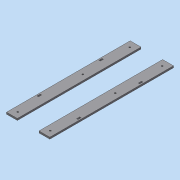
# Autodesk Inventor part: axis-holder_front-front
Saved by Autodesk Inventor 2016 SP1 (Build 200210100, 210)
## iProperties
Created: 2016-03-25
Part Number: axis-holder_front-front
Material: Generic
Document SubType Name: Modeling
Designer: Mohamed A.
Density: 1 g/cm^3
Appearance: Default
Author: Mohamed A.
Autodesk Inventor part; units mm, degrees
ref_plane "YZ Plane" through (0, 0, 0) normal (1, 0, 0) x (0, 1, 0)
ref_plane "XZ Plane" through (0, 0, 0) normal (0, 1, 0) x (-1, 0, 0)
ref_plane "XY Plane" through (0, 0, 0) normal (0, 0, 1) x (1, 0, 0)
sketch "Sketch1" plane through (0, 0, 0) normal (0, 0, 1) x (1, 0, 0)
  line L0 (-18.5, 195.95) -> (18.5, 195.95) construction
  line L1 (18.5, 195.95) -> (18.5, -15.45) construction
  line L2 (18.5, -15.45) -> (-18.5, -15.45) construction
  line L3 (-18.5, -15.45) -> (-18.5, 195.95) construction
  line L4 (-18.5, 195.95) -> (18.5, -15.45) construction
  line L5 (18.5, 195.95) -> (-18.5, -15.45) construction
  line L6 (18.5, 195.95) -> (37, 195.95)
  line L7 (37, 195.95) -> (37, -15.45)
  line L8 (37, -15.45) -> (18.5, -15.45)
  line L9 (18.5, -15.45) -> (18.5, 195.95)
  line L10 (0, -57.73) -> (0, 238.23) construction
  line L11 (-18.5, -15.45) -> (-37, -15.45)
  line L12 (-37, -15.45) -> (-37, 195.95)
  line L13 (-37, 195.95) -> (-18.5, 195.95)
  line L14 (-18.5, 195.95) -> (-18.5, -15.45)
  circle A0 centre (27.75, 185.95) radius 1.35
  circle A1 centre (-27.75, 185.95) radius 1.35
  circle A2 centre (27.75, -5.45) radius 1.35
  circle A3 centre (-27.75, -5.45) radius 1.35
  circle A4 centre (27.75, 105.7) radius 1.35
  circle A5 centre (-27.75, 105.7) radius 1.35
  point P0 (0, 0)
  point P1 (0, 90.25)
  point P2 (0, 90.25)
  dimension "d0" = 37
  dimension "d1" = 211.4
  dimension "d2" = 18.5
  dimension "d3" = 18.5
  dimension "d6" = 2.7
  dimension "d7" = 2.7
  dimension "d8" = 10
  dimension "d9" = 10
  dimension "d10" = 9.25
  dimension "d11" = 9.25
  dimension "d12" = 2.7
  dimension "d13" = 2.7
  dimension "d14" = 10
  dimension "d15" = 10
  dimension "d16" = 9.25
  dimension "d17" = 9.25
  dimension "d18" = 2.7
  dimension "d19" = 2.7
  dimension "d20" = 9.25
  dimension "d21" = 9.25
  dimension "d22" = 90.25
  dimension "d23" = 90.25
  constraints: 28 end point, 6 centre point, 6 parallel, 4 midpoint, 3 horizontal, 3 perpendicular, 2 collinear
  measures "d0" distance between parallel lines of L3 L1
  measures "d1" distance of L0.end L1.end
  measures "d2" distance of L0.end L6.end
  measures "d3" distance of L12.end L13.end
  measures "d6" diameter of A0
  measures "d7" diameter of A1
  measures "d8" distance from line of A0.centre L6
  measures "d9" distance from line of A1.centre L13
  measures "d10" distance from line of A1.centre L12
  measures "d11" distance from line of A0.centre L7
  measures "d12" diameter of A2
  measures "d13" diameter of A3
  measures "d14" distance from line of A2.centre L8
  measures "d15" distance from line of L11 A3.centre
  measures "d16" distance from line of A2.centre L7
  measures "d17" distance from line of L12 A3.centre
  measures "d18" diameter of A4
  measures "d19" diameter of A5
  measures "d20" distance from line of A4.centre L7
  measures "d21" distance from line of L12 A5.centre
  measures "d22" distance from line of L6 A4.centre
  measures "d23" distance from line of L13 A5.centre
extrude "Extrusion1" add sketch "Sketch1" along normal blind 3
sketch "Sketch2" plane through (0, 0, 3) normal (0, 0, 1) x (1, 0, 0)
  line L0 (35, 40.15) -> (32.5, 40.15) projected
  line L1 (32.5, 34.65) -> (35, 34.65) projected
  line L2 (-32.5, 40.15) -> (-35, 40.15) projected
  line L3 (-35, 34.65) -> (-32.5, 34.65) projected
  line L4 (-32.5, 140.4) -> (-35, 140.4) projected
  line L5 (-35, 145.8) -> (-32.5, 145.8) projected
  line L6 (32.5, 145.8) -> (35, 145.8) projected
  line L7 (32.5, 140.4) -> (35, 140.4) projected
  line L8 (35, 145.8) -> (35, 140.4)
  line L9 (37, -15.45) -> (37, 195.95) projected
  line L10 (32.5, 145.8) -> (32.5, 140.4)
  line L11 (-32.5, 145.8) -> (-32.5, 140.4)
  line L12 (-35, 145.8) -> (-35, 140.4)
  line L13 (-32.5, 40.15) -> (-32.5, 34.65)
  line L14 (-35, 40.15) -> (-35, 34.65)
  line L15 (35, 40.15) -> (35, 34.65)
  line L16 (32.5, 40.15) -> (32.5, 34.65)
  point P0 (0, 0)
  constraints: 16 end point, 8 parallel
extrude "Extrusion2" cut sketch "Sketch2" against normal blind 10
equation "\"d2\" = 0.5 * d0"
equation "\"d3\" = d2"
equation "\"d10\" = 0.5 * d3"
equation "\"d11\" = 0.5 * d2"
equation "\"d22\" = d23"
body "Solid1"
